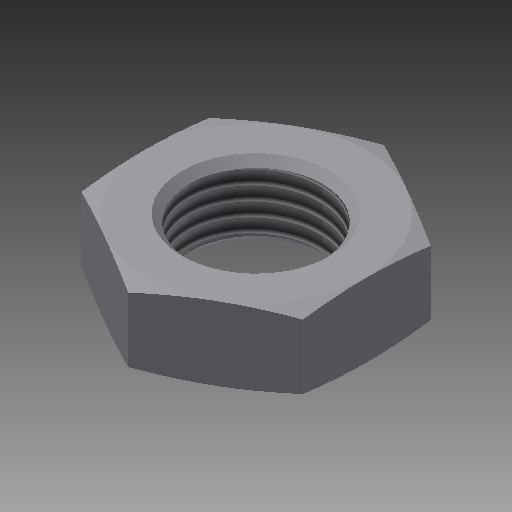
# Autodesk Inventor part: DIN-439-B - M16x1.5(F)
Saved by Autodesk Inventor 2018 (Build 220112000, 112)
## iProperties
Category: PARTsolutions
Company: FESTO
Created: 2019-05-10
Part Number: DIN-439-B - M16x1.5(F)
Material: Generic
Catalog Web Link: www.cadenas.de
Description: DIN-439 Form B-Hex nut
Vendor: FESTO
Document SubType Name: Modeling
Designer: psadmin
Manufacturer: FESTO
Mass: 2.64598 g
Surface Area: 16.3114 cm^2
Volume: 2.64598 cm^3
Density: 1 g/cm^3
Appearance: PSOLRGB-192-192-192
PSOL_IDENT_0: {$CADENAS_DATA\23d-libs\festo\zyl_zubeh\din_439_b\din_439_form_b.prj},190 {VTYP=3D},{NB=DIN-439-B -
PSOL_IDENT_1: M16x1.5(F)},{LINA=DIN-439-B - M16x1.5},{NN=DIN-439 Form B},{DATE=28.05.2015 11:05:12},{GEOMDATE=28.0
PSOL_IDENT_2: 5.2015 08:07:00},{VERSION=},{LINEID=170},{WBVAR=},{WBNUMERIC=}  {NB=DIN-439-B - M16x1.5(F)},{LINA=DI
PSOL_IDENT_3: N-439-B - M16x1.5},{KT=X},{IDNR=},{NENN=M16x1.5},{DG=16.000},{DK=14.376},{M=8.000},{S=24.000},{P=1.5
PSOL_IDENT_4: 00}
NN: DIN-439 Form B
NT: Hex nut
NB: DIN-439-B - M16x1.5(F)
NBSYN: DIN-439-B - $NENN.(F)
LINA: DIN-439-B - M16x1.5
ROWDESC: M16x1.5
NENN: M16x1.5
DG: 16
DK: 14.376
M: 8
S: 24
P: 1.5
SUPPLIER: FESTO
ARTICLENO: DIN-439-B - M16x1.5(F)
BOMINFO: DIN-439-B - M16x1.5
CREATOR: CADENAS GmbH
Title: DIN-439-B - M16x1.5
Author: Cadenas PARTsolutions
Comments: Hex nut
Autodesk Inventor part; units mm, degrees
sketch "Sketch_1" plane through (0, 0, 0) normal (0, 0, 1) x (1, 0, 0)
  line L0 (0, -8) -> (0, 0)
  line L1 (0, 0) -> (11.95, 0)
  line L2 (11.95, 0) -> (26.8782, -4)
  line L3 (26.8782, -4) -> (11.95, -8)
  line L4 (11.95, -8) -> (0, -8)
  line L5 (0, -8) -> (0, 0)
  constraints: 12 end point
revolve "Revolution1" add sketch "Sketch_1" angle 360 about axis through (0, -8, 0) along (0, 1, 0)
sketch "Sketch_2" plane through (0, 0, 0) normal (0, 1, 0) x (-1, 0, 0)
  line L0 (48, -48) -> (48, 48)
  line L1 (48, 48) -> (-48, 48)
  line L2 (-48, 48) -> (-48, -48)
  line L3 (-48, -48) -> (48, -48)
  line L4 (12, 6.9282) -> (0, 13.8564)
  line L5 (0, 13.8564) -> (-12, 6.9282)
  line L6 (-12, 6.9282) -> (-12, -6.9282)
  line L7 (-12, -6.9282) -> (0, -13.8564)
  line L8 (0, -13.8564) -> (12, -6.9282)
  line L9 (12, -6.9282) -> (12, 6.9282)
  constraints: 20 end point
extrude "Extrusion1" cut sketch "Sketch_2" along normal mid plane 18
sketch "Sketch_3" plane through (0, 0, 0) normal (0, 0, 1) x (1, 0, 0)
  line L0 (0, -8) -> (0, 0)
  line L1 (0, 0) -> (8, 0)
  line L2 (8, 0) -> (7.188, -0.812)
  line L3 (7.188, -0.812) -> (7.188, -7.188)
  line L4 (7.188, -7.188) -> (8, -8)
  line L5 (8, -8) -> (0, -8)
  line L6 (0, -8) -> (0, 0)
  constraints: 14 end point
revolve "Revolution2" cut sketch "Sketch_3" angle 360 about axis through (0, -8, 0) along (0, -1, 0)
thread "Thread1" size "M16x1.5" class "6H" standard "ISO Metric profile" full length
ref_plane "2CYL_XY" through (0, -4, 0) normal (0, 1, 0) x (1, 0, 0)
ref_plane "2CYL_YZ" through (0, -4, 0) normal (1, 0, 0) x (0, 0, -1)
ref_plane "2CYL_ZX" through (0, -4, 0) normal (0, 0, -1) x (0, 1, 0)
ref_plane "din439b_punkt_XY" through (0, 0, 0) normal (0, 1, 0) x (1, 0, 0)
ref_plane "din439b_punkt_YZ" through (0, 0, 0) normal (1, 0, 0) x (0, 0, -1)
ref_plane "din439b_punkt_ZX" through (0, 0, 0) normal (0, 0, -1) x (0, 1, 0)
body "Solid1"
